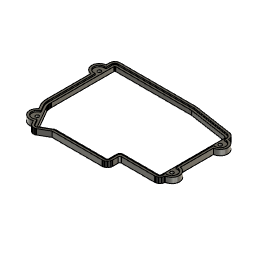
Lotus_case_v2 (Autodesk Fusion 360 design; units mm, degrees)
Autodesk Fusion 360 part; units mm, degrees
(part 1 of 2)
sketch "Sketch1" plane through (0, 0, 0) normal (0, 0, 1) x (1, 0, 0) in component "plate_left"
  circle A0 centre (76.6904, -49.9778) radius 4
  line L0 (80.5392, -30.7868) -> (81.5052, -30.6903)
  circle A1 centre (76.6904, -49.9778) radius 2
  line L1 (221.2947, -38.757) -> (223.044, -40.2889)
  circle A2 centre (86.1791, -132.9649) radius 2
  line L2 (81.5052, -30.6903) -> (172.0779, -30.687)
  line L3 (219.2863, -37.7893) -> (221.2947, -38.757)
  circle A3 centre (223.705, -53.9) radius 4
  circle A4 centre (223.705, -111.05) radius 2
  circle A5 centre (223.705, -111.05) radius 4
  circle A6 centre (223.705, -53.9) radius 2
  line L4 (172.0779, -30.687) -> (219.2863, -37.7893)
  line L5 (176.1036, -138.0502) -> (175.3059, -139.0179)
  line L6 (174.3382, -139.8156) -> (173.2321, -140.4142)
  line L7 (218.4, -126.194) -> (179.1936, -126.194)
  line L8 (99.2811, -148.0225) -> (98.1564, -148.3556)
  line L9 (224.5766, -121.0472) -> (224.2111, -122.2279)
  line L10 (76.6839, -118.0469) -> (76.2792, -116.505)
  line L11 (171.9999, -140.8) -> (170.9399, -140.905)
  line L12 (75.7005, -36.4881) -> (75.7987, -35.5252)
  line L13 (76.7158, -33.3442) -> (77.4564, -32.4462)
  line L14 (121.4, -62.05) -> (107.4, -62.05)
  line L15 (224.705, -119.9864) -> (224.5766, -121.0472)
  line L16 (173.2321, -140.4142) -> (171.9999, -140.8)
  line L17 (111.6629, -140.905) -> (99.9784, -147.6695)
  line L18 (76.2792, -116.505) -> (75.9418, -114.8181)
  line L19 (177.1936, -128.1938) -> (177.193, -134.6953)
  line L20 (99.9784, -147.6695) -> (99.2811, -148.0225)
  line L21 (75.7987, -35.5252) -> (76.1534, -34.3806)
  line L22 (77.4564, -32.4462) -> (78.3553, -31.7047)
  line L23 (121.4, -76.05) -> (121.4, -62.05)
  line L24 (130.85, -119.2) -> (116.85, -119.2)
  line L25 (223.044, -40.2889) -> (224.1387, -42.1727)
  line L26 (170.9399, -140.905) -> (111.6629, -140.905)
  line L27 (116.85, -119.2) -> (116.85, -133.2)
  line L28 (94.0822, -147.5328) -> (93.1049, -146.6975)
  line L29 (224.1387, -42.1727) -> (224.705, -44.1568)
  line L30 (107.4, -57) -> (121.4, -57)
  line L31 (121.4, -57) -> (121.4, -43)
  line L32 (176.7022, -136.9441) -> (176.1036, -138.0502)
  line L33 (75.7886, -113.0573) -> (75.7186, -112.1461)
  line L34 (75.7186, -112.1461) -> (75.6449, -110.7467)
  line L35 (116.85, -133.2) -> (130.85, -133.2)
  line L36 (107.4, -76.05) -> (121.4, -76.05)
  line L37 (98.23, -71.09) -> (98.23, -40.39)
  line L38 (223.6086, -123.3412) -> (222.8109, -124.3089)
  line L39 (177.082, -135.7313) -> (176.7022, -136.9441)
  line L40 (96.7866, -148.4476) -> (95.3567, -148.1592)
  line L41 (95.3567, -148.1592) -> (94.0822, -147.5328)
  line L42 (220.7348, -125.7064) -> (219.4745, -126.0997)
  line L43 (75.9418, -114.8181) -> (75.7886, -113.0573)
  line L44 (221.8432, -125.1066) -> (220.7348, -125.7064)
  line L45 (76.1534, -34.3806) -> (76.7158, -33.3442)
  line L46 (107.4, -43) -> (107.4, -57)
  line L47 (98.23, -40.39) -> (85.03, -40.39)
  line L48 (224.2111, -122.2279) -> (223.6086, -123.3412)
  line L49 (222.8109, -124.3089) -> (221.8432, -125.1066)
  line L50 (93.1049, -146.6975) -> (92.4734, -145.8895)
  line L51 (77.5111, -119.9268) -> (76.6839, -118.0469)
  line L52 (175.3059, -139.0179) -> (174.3382, -139.8156)
  line L53 (177.193, -134.6953) -> (177.082, -135.7313)
  line L54 (98.1564, -148.3556) -> (96.7866, -148.4476)
  line L55 (219.4745, -126.0997) -> (218.4, -126.194)
  line L56 (164.55, -97.75) -> (164.55, -111.75)
  line L57 (159.5, -77.31) -> (145.5, -77.31)
  line L58 (178.55, -54.6) -> (178.55, -40.6)
  line L59 (140.45, -73.65) -> (140.45, -59.65)
  line L60 (216.65, -99) -> (216.65, -85)
  line L61 (164.55, -111.75) -> (178.55, -111.75)
  line L62 (107.4, -100.15) -> (107.4, -114.15)
  line L63 (135.898, -117.828) -> (135.898, -131.828)
  line L64 (121.4, -114.15) -> (121.4, -100.15)
  line L65 (140.45, -40.6) -> (126.45, -40.6)
  line L66 (202.65, -99) -> (216.65, -99)
  line L67 (216.65, -60.9) -> (216.65, -46.9)
  line L68 (140.45, -78.7) -> (126.45, -78.7)
  line L69 (145.5, -72.26) -> (159.5, -72.26)
  line L70 (178.55, -111.75) -> (178.55, -97.75)
  line L71 (164.55, -73.65) -> (178.55, -73.65)
  line L72 (85.03, -71.09) -> (98.23, -71.09)
  line L73 (140.45, -54.6) -> (140.45, -40.6)
  line L74 (145.5, -91.31) -> (159.5, -91.31)
  line L75 (159.5, -72.26) -> (159.5, -58.26)
  line L76 (159.5, -58.26) -> (145.5, -58.26)
  line L77 (130.85, -133.2) -> (130.85, -119.2)
  line L78 (216.65, -46.9) -> (202.65, -46.9)
  line L79 (126.45, -40.6) -> (126.45, -54.6)
  line L80 (197.6, -78.45) -> (197.6, -64.45)
  line L81 (216.65, -85) -> (202.65, -85)
  line L82 (202.65, -85) -> (202.65, -99)
  line L83 (121.4, -43) -> (107.4, -43)
  line L84 (178.55, -40.6) -> (164.55, -40.6)
  line L85 (197.6, -102.55) -> (183.6, -102.55)
  line L86 (183.6, -102.55) -> (183.6, -116.55)
  line L87 (85.03, -40.39) -> (85.03, -71.09)
  line L88 (159.5, -91.31) -> (159.5, -77.31)
  line L89 (178.55, -73.65) -> (178.55, -59.65)
  line L90 (126.45, -92.7) -> (140.45, -92.7)
  line L91 (126.45, -54.6) -> (140.45, -54.6)
  line L92 (145.5, -58.26) -> (145.5, -72.26)
  line L93 (135.898, -131.828) -> (149.898, -131.828)
  line L94 (164.55, -40.6) -> (164.55, -54.6)
  line L95 (83.4748, -105.2852) -> (97.4748, -105.2852)
  line L96 (202.65, -60.9) -> (216.65, -60.9)
  line L97 (183.6, -83.5) -> (183.6, -97.5)
  line L98 (140.45, -59.65) -> (126.45, -59.65)
  line L99 (164.55, -59.65) -> (164.55, -73.65)
  line L100 (145.5, -77.31) -> (145.5, -91.31)
  line L101 (183.6, -116.55) -> (197.6, -116.55)
  line L102 (183.6, -78.45) -> (197.6, -78.45)
  line L103 (126.45, -59.65) -> (126.45, -73.65)
  line L104 (183.6, -97.5) -> (197.6, -97.5)
  line L105 (197.6, -64.45) -> (183.6, -64.45)
  line L106 (97.4748, -105.2852) -> (97.4748, -91.2851)
  line L107 (197.6, -83.5) -> (183.6, -83.5)
  line L108 (83.4748, -91.2851) -> (83.4748, -105.2852)
  line L109 (183.6, -64.45) -> (183.6, -78.45)
  line L110 (178.55, -59.65) -> (164.55, -59.65)
  line L111 (140.45, -92.7) -> (140.45, -78.7)
  line L112 (197.6, -116.55) -> (197.6, -102.55)
  line L113 (126.45, -73.65) -> (140.45, -73.65)
  line L114 (149.898, -131.828) -> (149.898, -117.828)
  line L115 (107.4, -62.05) -> (107.4, -76.05)
  line L116 (149.898, -117.828) -> (135.898, -117.828)
  line L117 (202.65, -46.9) -> (202.65, -60.9)
  line L118 (178.55, -97.75) -> (164.55, -97.75)
  line L119 (107.4, -114.15) -> (121.4, -114.15)
  line L120 (121.4, -100.15) -> (107.4, -100.15)
  line L121 (197.6, -97.5) -> (197.6, -83.5)
  line L122 (145.5, -96.36) -> (145.5, -110.36)
  line L123 (164.55, -54.6) -> (178.55, -54.6)
  line L124 (145.5, -110.36) -> (159.5, -110.36)
  line L125 (126.45, -78.7) -> (126.45, -92.7)
  line L126 (79.3908, -31.1434) -> (80.5392, -30.7868)
  line L127 (78.3553, -31.7047) -> (79.3908, -31.1434)
  arc A7 (75.6971, -41.0327) -> (75.6837, -58.9213) centre (76.6904, -49.9778) ccw
  arc A8 (224.704, -119.9944) -> (224.705, -102.1057) centre (223.705, -111.05) ccw
  arc A9 (80.8467, -125.7147) -> (89.7788, -141.2137) centre (86.1791, -132.9649) ccw
  arc A10 (224.705, -62.8443) -> (224.705, -44.9557) centre (223.705, -53.9) ccw
  circle A11 centre (86.1791, -132.9649) radius 4
  line L128 (144.5, -92.31) -> (160.5, -92.31)
  line L129 (182.6, -98.5) -> (198.6, -98.5)
  line L130 (125.45, -93.7) -> (141.45, -93.7)
  line L131 (163.55, -58.65) -> (163.55, -74.65)
  line L132 (141.45, -77.7) -> (125.45, -77.7)
  line L133 (179.55, -77.7) -> (163.55, -77.7)
  line L134 (179.55, -58.65) -> (163.55, -58.65)
  line L135 (125.45, -77.7) -> (125.45, -93.7)
  line L136 (217.65, -100) -> (217.65, -84)
  line L137 (198.6, -63.45) -> (182.6, -63.45)
  line L138 (144.5, -76.31) -> (144.5, -92.31)
  line L139 (182.6, -79.45) -> (198.6, -79.45)
  line L140 (198.6, -82.5) -> (182.6, -82.5)
  line L141 (201.65, -80.95) -> (217.65, -80.95)
  line L142 (198.6, -79.45) -> (198.6, -63.45)
  line L143 (217.65, -119.05) -> (217.65, -103.05)
  line L144 (201.65, -103.05) -> (201.65, -119.05)
  line L145 (198.6, -101.55) -> (182.6, -101.55)
  line L146 (217.65, -64.95) -> (201.65, -64.95)
  line L147 (106.4, -96.1) -> (122.4, -96.1)
  line L148 (201.65, -84) -> (201.65, -100)
  line L149 (163.55, -74.65) -> (179.55, -74.65)
  line L150 (163.55, -93.7) -> (179.55, -93.7)
  line L151 (217.65, -80.95) -> (217.65, -64.95)
  line L152 (163.55, -112.75) -> (179.55, -112.75)
  line L153 (179.55, -74.65) -> (179.55, -58.65)
  line L154 (160.5, -92.31) -> (160.5, -76.31)
  line L155 (144.5, -95.36) -> (144.5, -111.36)
  line L156 (163.55, -96.75) -> (163.55, -112.75)
  line L157 (141.45, -96.75) -> (125.45, -96.75)
  line L158 (106.4, -80.1) -> (106.4, -96.1)
  line L159 (182.6, -63.45) -> (182.6, -79.45)
  line L160 (144.5, -111.36) -> (160.5, -111.36)
  line L161 (198.6, -117.55) -> (198.6, -101.55)
  line L162 (217.65, -103.05) -> (201.65, -103.05)
  line L163 (125.45, -96.75) -> (125.45, -112.75)
  line L164 (125.45, -112.75) -> (141.45, -112.75)
  line L165 (201.65, -119.05) -> (217.65, -119.05)
  line L166 (160.5, -76.31) -> (144.5, -76.31)
  line L167 (160.5, -73.26) -> (160.5, -57.26)
  line L168 (201.65, -100) -> (217.65, -100)
  line L169 (106.4, -115.15) -> (122.4, -115.15)
  line L170 (198.6, -98.5) -> (198.6, -82.5)
  line L171 (217.65, -84) -> (201.65, -84)
  line L172 (179.55, -96.75) -> (163.55, -96.75)
  line L173 (122.4, -80.1) -> (106.4, -80.1)
  line L174 (182.6, -117.55) -> (198.6, -117.55)
  line L175 (122.4, -115.15) -> (122.4, -99.15)
  line L176 (97.4748, -91.2851) -> (83.4748, -91.2851)
  line L177 (80.7003, -36.7444) -> (80.7223, -36.5288)
  line L178 (80.645, -110.617) -> (80.7003, -36.7444)
  line L179 (97.4269, -143.357) -> (97.2682, -143.404)
  line L180 (164.55, -92.7) -> (178.55, -92.7)
  line L181 (80.7834, -36.3316) -> (80.8802, -36.1532)
  line L182 (219.705, -119.685) -> (219.667, -119.999)
  line L183 (159.5, -110.36) -> (159.5, -96.36)
  line L184 (219.442, -120.535) -> (219.259, -120.757)
  line L185 (80.7223, -36.5288) -> (80.7834, -36.3316)
  line L186 (173.244, -122.218) -> (172.817, -122.736)
  line L187 (219.58, -120.28) -> (219.442, -120.535)
  line L188 (178.55, -92.7) -> (178.55, -78.7)
  line L189 (171.704, -35.687) -> (217.796, -42.6214)
  line L190 (97.5948, -143.272) -> (97.4269, -143.357)
  line L191 (140.45, -97.75) -> (126.45, -97.75)
  line L192 (97.2682, -143.404) -> (97.1193, -143.414)
  line L193 (171.532, -135.649) -> (171.277, -135.787)
  line L194 (96.8523, -143.323) -> (96.7353, -143.223)
  line L195 (81.153, -115.379) -> (80.899, -114.109)
  line L196 (81.5392, -35.7118) -> (81.7544, -35.6903)
  line L197 (80.899, -114.109) -> (80.772, -112.649)
  line L198 (80.8802, -36.1532) -> (81.0083, -35.9979)
  line L199 (219.133, -43.5102) -> (219.502, -44.1452)
  line L200 (171.277, -135.787) -> (170.996, -135.875)
  line L201 (140.45, -111.75) -> (140.45, -97.75)
  line L202 (218.512, -42.9664) -> (219.133, -43.5102)
  line L203 (217.796, -42.6214) -> (218.512, -42.9664)
  line L204 (126.45, -97.75) -> (126.45, -111.75)
  line L205 (80.7085, -111.823) -> (80.645, -110.617)
  line L206 (81.0083, -35.9979) -> (81.1637, -35.8697)
  line L207 (219.705, -44.8564) -> (219.705, -119.685)
  line L208 (96.9805, -143.386) -> (96.8523, -143.323)
  line L209 (170.693, -135.905) -> (110.32, -135.905)
  line L210 (219.667, -119.999) -> (219.58, -120.28)
  line L211 (219.037, -120.94) -> (218.782, -121.078)
  line L212 (171.937, -135.244) -> (171.754, -135.466)
  line L213 (97.1193, -143.414) -> (96.9805, -143.386)
  line L214 (80.772, -112.649) -> (80.7085, -111.823)
  line L215 (81.9785, -117.665) -> (81.4197, -116.395)
  line L216 (96.7353, -143.223) -> (96.6298, -143.088)
  line L217 (178.55, -78.7) -> (164.55, -78.7)
  line L218 (216.65, -79.95) -> (216.65, -65.95)
  line L219 (81.1637, -35.8697) -> (81.3421, -35.773)
  line L220 (218.782, -121.078) -> (218.5, -121.166)
  line L221 (218.5, -121.166) -> (218.181, -121.194)
  line L222 (175.719, -121.194) -> (175.014, -121.265)
  line L223 (96.6298, -143.088) -> (81.9785, -117.665)
  line L224 (171.754, -135.466) -> (171.532, -135.649)
  line L225 (175.014, -121.265) -> (174.356, -121.468)
  line L226 (218.181, -121.194) -> (175.719, -121.194)
  line L227 (81.3421, -35.773) -> (81.5392, -35.7118)
  line L228 (219.259, -120.757) -> (219.037, -120.94)
  line L229 (110.32, -135.905) -> (97.5948, -143.272)
  line L230 (202.65, -79.95) -> (216.65, -79.95)
  line L231 (219.502, -44.1452) -> (219.705, -44.8564)
  line L232 (126.45, -111.75) -> (140.45, -111.75)
  line L233 (170.996, -135.875) -> (170.693, -135.905)
  line L234 (173.762, -121.791) -> (173.244, -122.218)
  line L235 (174.356, -121.468) -> (173.762, -121.791)
  line L236 (202.65, -65.95) -> (202.65, -79.95)
  line L237 (164.55, -78.7) -> (164.55, -92.7)
  line L238 (216.65, -65.95) -> (202.65, -65.95)
  line L239 (159.5, -96.36) -> (145.5, -96.36)
  line L240 (81.7544, -35.6903) -> (171.704, -35.687)
  line L241 (81.4197, -116.395) -> (81.153, -115.379)
  line L242 (163.55, -55.6) -> (179.55, -55.6)
  line L243 (107.4, -81.1) -> (107.4, -95.1)
  line L244 (106.4, -42) -> (106.4, -58)
  line L245 (145.5, -39.21) -> (145.5, -53.21)
  line L246 (217.65, -61.9) -> (217.65, -45.9)
  line L247 (95.609, -135.6097) -> (107.7334, -128.6097)
  line L248 (159.5, -53.21) -> (159.5, -39.21)
  line L249 (141.45, -58.65) -> (125.45, -58.65)
  line L250 (160.5, -38.21) -> (144.5, -38.21)
  line L251 (172.817, -122.736) -> (172.494, -123.331)
  line L252 (179.55, -39.6) -> (163.55, -39.6)
  line L253 (182.6, -60.4) -> (198.6, -60.4)
  line L254 (198.6, -60.4) -> (198.6, -44.4)
  line L255 (122.4, -58) -> (122.4, -42)
  line L256 (172.075, -134.989) -> (171.937, -135.244)
  line L257 (125.45, -74.65) -> (141.45, -74.65)
  line L258 (183.6, -59.4) -> (197.6, -59.4)
  line L259 (125.45, -58.65) -> (125.45, -74.65)
  line L260 (144.5, -38.21) -> (144.5, -54.21)
  line L261 (172.29, -123.988) -> (172.194, -124.696)
  line L262 (100.7334, -116.4853) -> (88.609, -123.4853)
  line L263 (172.494, -123.331) -> (172.29, -123.988)
  line L264 (201.65, -45.9) -> (201.65, -61.9)
  line L265 (144.5, -73.26) -> (160.5, -73.26)
  line L266 (122.4, -61.05) -> (106.4, -61.05)
  line L267 (106.4, -61.05) -> (106.4, -77.05)
  line L268 (216.65, -118.05) -> (216.65, -104.05)
  line L269 (122.4, -42) -> (106.4, -42)
  line L270 (121.4, -81.1) -> (107.4, -81.1)
  line L271 (197.6, -45.4) -> (183.6, -45.4)
  line L272 (125.45, -55.6) -> (141.45, -55.6)
  line L273 (183.6, -45.4) -> (183.6, -59.4)
  line L274 (160.5, -54.21) -> (160.5, -38.21)
  line L275 (154.95, -130.8) -> (168.95, -130.8)
  line L276 (197.6, -59.4) -> (197.6, -45.4)
  line L277 (107.7334, -128.6097) -> (100.7334, -116.4853)
  line L278 (121.4, -95.1) -> (121.4, -81.1)
  line L279 (106.4, -58) -> (122.4, -58)
  line L280 (202.65, -118.05) -> (216.65, -118.05)
  line L281 (216.65, -104.05) -> (202.65, -104.05)
  line L282 (141.45, -39.6) -> (125.45, -39.6)
  line L283 (125.45, -39.6) -> (125.45, -55.6)
  line L284 (202.65, -104.05) -> (202.65, -118.05)
  line L285 (172.194, -124.696) -> (172.193, -134.428)
  line L286 (122.4, -77.05) -> (122.4, -61.05)
  line L287 (163.55, -39.6) -> (163.55, -55.6)
  line L288 (179.55, -55.6) -> (179.55, -39.6)
  line L289 (217.65, -45.9) -> (201.65, -45.9)
  line L290 (141.45, -55.6) -> (141.45, -39.6)
  line L291 (198.6, -44.4) -> (182.6, -44.4)
  line L292 (141.45, -74.65) -> (141.45, -58.65)
  line L293 (168.95, -130.8) -> (168.95, -116.8)
  line L294 (145.5, -53.21) -> (159.5, -53.21)
  line L295 (154.95, -116.8) -> (154.95, -130.8)
  line L296 (168.95, -116.8) -> (154.95, -116.8)
  line L297 (182.6, -44.4) -> (182.6, -60.4)
  line L298 (144.5, -54.21) -> (160.5, -54.21)
  line L299 (122.4, -96.1) -> (122.4, -80.1)
  line L300 (159.5, -39.21) -> (145.5, -39.21)
  line L301 (88.609, -123.4853) -> (95.609, -135.6097)
  line L302 (172.193, -134.428) -> (172.163, -134.708)
  line L303 (106.4, -77.05) -> (122.4, -77.05)
  line L304 (201.65, -61.9) -> (217.65, -61.9)
  line L305 (107.4, -95.1) -> (121.4, -95.1)
  line L306 (172.163, -134.708) -> (172.075, -134.989)
  line L307 (160.5, -95.36) -> (144.5, -95.36)
  line L308 (141.45, -112.75) -> (141.45, -96.75)
  line L309 (122.4, -99.15) -> (106.4, -99.15)
  line L310 (160.5, -57.26) -> (144.5, -57.26)
  line L311 (201.65, -64.95) -> (201.65, -80.95)
  line L312 (179.55, -93.7) -> (179.55, -77.7)
  line L313 (179.55, -112.75) -> (179.55, -96.75)
  line L314 (144.5, -57.26) -> (144.5, -73.26)
  line L315 (106.4, -99.15) -> (106.4, -115.15)
  line L316 (182.6, -82.5) -> (182.6, -98.5)
  line L317 (182.6, -101.55) -> (182.6, -117.55)
  line L318 (163.55, -77.7) -> (163.55, -93.7)
  line L319 (141.45, -93.7) -> (141.45, -77.7)
  line L320 (82.4748, -106.2852) -> (98.4748, -106.2852)
  line L321 (160.5, -111.36) -> (160.5, -95.36)
  line L322 (95.23, -68.09) -> (95.23, -43.39)
  line L323 (88.03, -43.39) -> (88.03, -68.09)
  line L324 (169.95, -131.8) -> (169.95, -115.8)
  line L325 (82.4748, -90.2851) -> (82.4748, -106.2852)
  line L326 (131.85, -134.2) -> (131.85, -118.2)
  line L327 (115.85, -134.2) -> (131.85, -134.2)
  line L328 (115.85, -118.2) -> (115.85, -134.2)
  line L329 (87.243, -123.1193) -> (95.243, -136.9757)
  line L330 (150.898, -132.828) -> (150.898, -116.828)
  line L331 (95.243, -136.9757) -> (109.0994, -128.9757)
  line L332 (150.898, -116.828) -> (134.898, -116.828)
  line L333 (98.4748, -90.2851) -> (82.4748, -90.2851)
  line L334 (131.85, -118.2) -> (115.85, -118.2)
  line L335 (98.4748, -106.2852) -> (98.4748, -90.2851)
  line L336 (169.95, -115.8) -> (153.95, -115.8)
  line L337 (153.95, -131.8) -> (169.95, -131.8)
  line L338 (153.95, -115.8) -> (153.95, -131.8)
  line L339 (88.03, -68.09) -> (95.23, -68.09)
  line L340 (134.898, -132.828) -> (150.898, -132.828)
  line L341 (101.0994, -115.1193) -> (87.243, -123.1193)
  line L342 (134.898, -116.828) -> (134.898, -132.828)
  line L343 (109.0994, -128.9757) -> (101.0994, -115.1193)
  line L344 (95.23, -43.39) -> (88.03, -43.39)
  line L345 (218.5412, -40.2054) -> (219.9033, -40.8617)
  line L346 (219.9033, -40.8617) -> (221.0885, -41.8996)
  line L347 (221.0885, -41.8996) -> (221.8203, -43.1589)
  line L348 (221.8203, -43.1589) -> (222.205, -44.5066)
  line L349 (222.205, -119.8357) -> (222.1218, -120.5231)
  line L350 (222.1218, -120.5231) -> (221.8955, -121.2539)
  line L351 (221.8955, -121.2539) -> (221.5253, -121.9381)
  line L352 (221.5253, -121.9381) -> (221.0349, -122.5329)
  line L353 (221.0349, -122.5329) -> (220.4401, -123.0233)
  line L354 (220.4401, -123.0233) -> (219.7584, -123.3922)
  line L355 (219.7584, -123.3922) -> (218.9873, -123.6328)
  line L356 (218.9873, -123.6328) -> (218.2905, -123.694)
  line L357 (218.2905, -123.694) -> (177.6938, -123.694)
  line L358 (174.6938, -126.6937) -> (174.693, -134.5617)
  line L359 (174.693, -134.5617) -> (174.6225, -135.2197)
  line L360 (174.6225, -135.2197) -> (174.3886, -135.9665)
  line L361 (174.3886, -135.9665) -> (174.0203, -136.6471)
  line L362 (174.0203, -136.6471) -> (173.5299, -137.2419)
  line L363 (173.5299, -137.2419) -> (172.9351, -137.7323)
  line L364 (172.9351, -137.7323) -> (172.2545, -138.1006)
  line L365 (172.2545, -138.1006) -> (171.498, -138.3375)
  line L366 (171.498, -138.3375) -> (170.8165, -138.405)
  line L367 (170.8165, -138.405) -> (110.9915, -138.405)
  line L368 (110.9915, -138.405) -> (98.7866, -145.4708)
  line L369 (98.7866, -145.4708) -> (98.354, -145.6898)
  line L370 (98.354, -145.6898) -> (97.7123, -145.8798)
  line L371 (97.7123, -145.8798) -> (96.953, -145.9308)
  line L372 (96.953, -145.9308) -> (96.1686, -145.7726)
  line L373 (96.1686, -145.7726) -> (95.4672, -145.4279)
  line L374 (95.4672, -145.4279) -> (94.9201, -144.9603)
  line L375 (94.9201, -144.9603) -> (94.5516, -144.4887)
  line L376 (79.7448, -118.7959) -> (79.0518, -117.2209)
  line L377 (79.0518, -117.2209) -> (78.7161, -115.942)
  line L378 (78.7161, -115.942) -> (78.4204, -114.4636)
  line L379 (78.4204, -114.4636) -> (78.2803, -112.8531)
  line L380 (78.2803, -112.8531) -> (78.2135, -111.9846)
  line L381 (78.2135, -111.9846) -> (78.145, -110.6818)
  line L382 (78.2004, -36.6162) -> (78.2605, -36.027)
  line L383 (78.2605, -36.027) -> (78.4684, -35.3561)
  line L384 (78.4684, -35.3561) -> (78.798, -34.7487)
  line L385 (78.798, -34.7487) -> (79.2324, -34.2221)
  line L386 (79.2324, -34.2221) -> (79.7595, -33.7872)
  line L387 (79.7595, -33.7872) -> (80.3665, -33.4582)
  line L388 (80.3665, -33.4582) -> (81.0392, -33.2493)
  line L389 (81.0392, -33.2493) -> (81.6298, -33.1903)
  line L390 (81.6298, -33.1903) -> (171.891, -33.187)
  line L391 (171.891, -33.187) -> (218.5412, -40.2054)
  arc A12 (78.1951, -43.6543) -> (78.1857, -56.3034) centre (76.6904, -49.9778) ccw
  line L392 (78.1951, -43.6543) -> (78.2004, -36.6162)
  line L393 (75.6971, -41.0327) -> (75.7005, -36.4881)
  line L394 (78.145, -110.6818) -> (78.1857, -56.3034)
  line L395 (75.6449, -110.7467) -> (75.6837, -58.9213)
  arc A13 (84.3208, -126.7362) -> (90.6367, -137.6956) centre (86.1791, -132.9649) ccw
  line L396 (94.5516, -144.4887) -> (90.6367, -137.6956)
  line L397 (84.3208, -126.7362) -> (79.7448, -118.7959)
  line L398 (80.8467, -125.7147) -> (77.5111, -119.9268)
  line L399 (92.4734, -145.8895) -> (89.7788, -141.2137)
  arc A14 (222.205, -117.3746) -> (222.205, -104.7254) centre (223.705, -111.05) ccw
  line L400 (222.205, -117.3746) -> (222.205, -119.8357)
  line L401 (224.705, -62.8443) -> (224.705, -102.1057)
  line L402 (224.705, -44.1568) -> (224.705, -44.9557)
  arc A15 (222.205, -60.2246) -> (222.205, -47.5754) centre (223.705, -53.9) ccw
  line L403 (222.205, -60.2246) -> (222.205, -104.7254)
  line L404 (222.205, -44.5066) -> (222.205, -47.5754)
  arc A16 (179.1936, -126.194) -> (177.1936, -128.1938) centre (179.1936, -128.194) ccw
  arc A17 (177.6938, -123.694) -> (174.6938, -126.6937) centre (177.6938, -126.694) ccw
  dimension "d6" = 13
  dimension "d7" = 13
  dimension "d8" = 13
  dimension "d9" = 13
  dimension "d10" = 2
  dimension "d11" = 3
  constraint concentric A1 A12
  constraint concentric A11 A13
  constraint concentric A5 A14
  constraint concentric A10 A15
  constraint coincident A12.start L394
  constraint collinear L392 L394
  constraint collinear L393 L395
  constraint coincident A13.start L396
  constraint collinear L396 L397
  constraint collinear L398 L399
  constraint coincident A14.start L404
  constraint collinear L400 L404
  constraint collinear L401 L402
  constraint coincident A15.start L404
  constraint collinear L403 L404
  constraint tangent L19 A16
  constraint tangent L7 A16
  constraint tangent L358 A17
  constraint tangent L357 A17
  measures "d6" diameter of A12
  measures "d7" diameter of A13
  measures "d8" diameter of A14
  measures "d9" diameter of A15
  measures "d10" radius of A16
  measures "d11" radius of A17
form "Form1" [no effect] in component "plate_left"
extrude "Extrude1" add sketch "Sketch1" along normal blind 3 contours A0 | L177 L178 L179 L181 L182 L184 L185 L186 L187 L189 L190 L192 L193 L194 L195 L196 L197 L198 L199 L200 L202 L203 L205 L206 L207 L208 L209 L210 L211 L212 L213 L214 L215 L216 L219 L220 L221 L222 L223 L224 L225 L226 L227 L228 L229 L231 L233 L234 L235 L240 L241 L251 L256 L261 L263 L285 L302 L306 | A3 | A5 | A11 | L0 L1 L2 L3 L4 L5 L6 L7 L8 L9 L10 L11 L12 L13 L15 L16 L17 L18 L19 L20 L21 L22 L25 L26 L28 L29 L32 L33 L34 L38 L39 L40 L41 L42 L43 L44 L45 L48 L49 L50 L51 L52 L53 L54 L55 L126 L127 A7 A8 A9 A10 L393 L395 L398 L399 L401 L402 A16 | L345 L346 L347 L348 L349 L350 L351 L352 L353 L354 L355 L356 L357 L358 L359 L360 L361 L362 L363 L364 L365 L366 L367 L368 L369 L370 L371 L372 L373 L374 L375 L376 L377 L378 L379 L380 L381 L382 L383 L384 L385 L386 L387 L388 L389 L390 L391 A12 L392 L394 A13 L396 L397 A14 L400 A15 L403 L404 A17 makes body 1 in component "plate_left"
extrude "Extrude2" add sketch "Sketch1" along normal blind 1.5 contours L37 L47 L72 L87 | L128 L138 L154 L166 | L129 L140 L170 L316 | L130 L132 L135 L319 | L131 L134 L149 L153 | L133 L150 L312 L318 | L136 L148 L168 L171 | L137 L139 L142 L159 | L141 L146 L151 L311 | L143 L144 L162 L165 | L145 L161 L174 L317 | L147 L158 L173 L299 | L152 L156 L172 L313 | L155 L160 L307 L321 | L157 L163 L164 L308 | L167 L265 L310 L314 | L169 L175 L309 L315 | L242 L252 L287 L288 | L244 L255 L269 L279 | L246 L264 L289 L304 | L249 L257 L259 L292 | L250 L260 L274 L298 | L253 L254 L291 L297 | L266 L267 L286 L303 | L272 L282 L283 L290 | L320 L325 L333 L335 | L324 L336 L337 L338 | L326 L327 L328 L334 | L329 L331 L341 L343 | L330 L332 L340 L342 bodies 1 in component "plate_left"
extrude "Extrude3" cut sketch "Sketch1" along normal blind 3 contours L0 L1 L2 L3 L4 L5 L6 L7 L8 L9 L10 L11 L12 L13 L15 L16 L17 L18 L19 L20 L21 L22 L25 L26 L28 L29 L32 L33 L34 L38 L39 L40 L41 L42 L43 L44 L45 L48 L49 L50 L51 L52 L53 L54 L55 L126 L127 A7 A8 A9 A10 L393 L395 L398 L399 L401 L402 A16 bodies 1 in component "plate_left"
sketch "clean_plate_v4.1" plane through (0, 0, 0) normal (0, 0, 1) x (1, 0, 0) in component "bottom_right"
  line L0 (78.2605, -36.027) -> (78.4684, -35.3561)
  line L1 (81.0392, -33.2493) -> (81.6298, -33.1903)
  line L2 (78.4684, -35.3561) -> (78.798, -34.7487)
  line L3 (171.891, -33.187) -> (218.5412, -40.2054)
  line L4 (78.2004, -36.6162) -> (78.2605, -36.027)
  line L5 (78.798, -34.7487) -> (79.2324, -34.2221)
  line L6 (75.6449, -110.7467) -> (75.6837, -58.9213)
  line L7 (224.705, -44.1568) -> (224.705, -44.9557)
  arc A0 (78.1857, -56.3034) -> (78.1951, -43.6543) centre (76.6904, -49.9778) cw
  line L8 (82.4748, -106.2852) -> (98.4748, -106.2852)
  line L9 (98.4748, -90.2851) -> (82.4748, -90.2851)
  line L10 (168.95, -116.8) -> (154.95, -116.8)
  line L11 (125.45, -39.6) -> (125.45, -55.6)
  line L12 (154.95, -130.8) -> (168.95, -130.8)
  line L13 (95.23, -43.39) -> (88.03, -43.39)
  line L14 (95.23, -68.09) -> (95.23, -43.39)
  line L15 (98.4748, -106.2852) -> (98.4748, -90.2851)
  line L16 (202.65, -104.05) -> (202.65, -118.05)
  line L17 (154.95, -116.8) -> (154.95, -130.8)
  line L18 (216.65, -118.05) -> (216.65, -104.05)
  line L19 (216.65, -104.05) -> (202.65, -104.05)
  line L20 (122.4, -77.05) -> (122.4, -61.05)
  line L21 (168.95, -130.8) -> (168.95, -116.8)
  line L22 (202.65, -118.05) -> (216.65, -118.05)
  line L23 (141.45, -39.6) -> (125.45, -39.6)
  line L24 (141.45, -55.6) -> (141.45, -39.6)
  line L25 (125.45, -55.6) -> (141.45, -55.6)
  line L26 (216.65, -79.95) -> (216.65, -65.95)
  line L27 (82.4748, -90.2851) -> (82.4748, -106.2852)
  line L28 (80.8467, -125.7147) -> (77.5111, -119.9268)
  line L29 (78.1951, -43.6543) -> (78.2004, -36.6162)
  line L30 (79.7595, -33.7872) -> (80.3665, -33.4582)
  line L31 (224.705, -62.8443) -> (224.705, -102.1057)
  line L32 (75.6971, -41.0327) -> (75.7005, -36.4881)
  line L33 (171.498, -138.3375) -> (170.8165, -138.405)
  line L34 (170.8165, -138.405) -> (110.9915, -138.405)
  line L35 (87.243, -123.1193) -> (95.243, -136.9757)
  line L36 (222.205, -60.2246) -> (222.205, -104.7254)
  line L37 (115.85, -118.2) -> (115.85, -134.2)
  line L38 (150.898, -132.828) -> (150.898, -116.828)
  line L39 (174.0203, -136.6471) -> (173.5299, -137.2419)
  line L40 (78.145, -110.6818) -> (78.1857, -56.3034)
  line L41 (92.4734, -145.8895) -> (89.7788, -141.2137)
  line L42 (79.2324, -34.2221) -> (79.7595, -33.7872)
  arc A1 (179.1936, -126.194) -> (177.1936, -128.1938) centre (179.1936, -128.194) ccw
  line L43 (80.3665, -33.4582) -> (81.0392, -33.2493)
  line L44 (81.6298, -33.1903) -> (171.891, -33.187)
  line L45 (131.85, -118.2) -> (115.85, -118.2)
  line L46 (222.205, -119.8357) -> (222.1218, -120.5231)
  line L47 (169.95, -115.8) -> (153.95, -115.8)
  line L48 (153.95, -131.8) -> (169.95, -131.8)
  line L49 (115.85, -134.2) -> (131.85, -134.2)
  line L50 (222.205, -117.3746) -> (222.205, -119.8357)
  line L51 (220.4401, -123.0233) -> (219.7584, -123.3922)
  line L52 (219.7584, -123.3922) -> (218.9873, -123.6328)
  line L53 (174.6225, -135.2197) -> (174.3886, -135.9665)
  line L54 (221.8203, -43.1589) -> (222.205, -44.5066)
  arc A2 (222.205, -104.7254) -> (222.205, -117.3746) centre (223.705, -111.05) cw
  line L55 (134.898, -116.828) -> (134.898, -132.828)
  line L56 (169.95, -131.8) -> (169.95, -115.8)
  line L57 (163.55, -77.7) -> (163.55, -93.7)
  line L58 (197.6, -83.5) -> (183.6, -83.5)
  line L59 (197.6, -102.55) -> (183.6, -102.55)
  line L60 (141.45, -77.7) -> (125.45, -77.7)
  line L61 (198.6, -98.5) -> (198.6, -82.5)
  line L62 (179.55, -58.65) -> (163.55, -58.65)
  line L63 (183.6, -78.45) -> (197.6, -78.45)
  line L64 (78.3553, -31.7047) -> (79.3908, -31.1434)
  line L65 (198.6, -82.5) -> (182.6, -82.5)
  line L66 (159.5, -96.36) -> (145.5, -96.36)
  line L67 (217.65, -84) -> (201.65, -84)
  line L68 (125.45, -93.7) -> (141.45, -93.7)
  line L69 (163.55, -74.65) -> (179.55, -74.65)
  line L70 (201.65, -100) -> (217.65, -100)
  circle A3 centre (86.1791, -132.9649) radius 4
  line L71 (182.6, -63.45) -> (182.6, -79.45)
  line L72 (79.3908, -31.1434) -> (80.5392, -30.7868)
  line L73 (145.5, -110.36) -> (159.5, -110.36)
  line L74 (179.55, -93.7) -> (179.55, -77.7)
  line L75 (198.6, -79.45) -> (198.6, -63.45)
  line L76 (217.65, -80.95) -> (217.65, -64.95)
  line L77 (179.55, -77.7) -> (163.55, -77.7)
  line L78 (217.65, -64.95) -> (201.65, -64.95)
  line L79 (201.65, -84) -> (201.65, -100)
  line L80 (179.55, -74.65) -> (179.55, -58.65)
  line L81 (183.6, -97.5) -> (197.6, -97.5)
  line L82 (159.5, -110.36) -> (159.5, -96.36)
  line L83 (201.65, -64.95) -> (201.65, -80.95)
  line L84 (217.65, -103.05) -> (201.65, -103.05)
  line L85 (217.65, -100) -> (217.65, -84)
  line L86 (201.65, -103.05) -> (201.65, -119.05)
  line L87 (201.65, -119.05) -> (217.65, -119.05)
  line L88 (198.6, -63.45) -> (182.6, -63.45)
  line L89 (198.6, -101.55) -> (182.6, -101.55)
  line L90 (217.65, -119.05) -> (217.65, -103.05)
  line L91 (125.45, -77.7) -> (125.45, -93.7)
  line L92 (182.6, -101.55) -> (182.6, -117.55)
  arc A4 (224.705, -62.8443) -> (224.705, -44.9557) centre (223.705, -53.9) ccw
  line L93 (163.55, -55.6) -> (179.55, -55.6)
  line L94 (179.55, -39.6) -> (163.55, -39.6)
  line L95 (144.5, -54.21) -> (160.5, -54.21)
  line L96 (88.609, -123.4853) -> (95.609, -135.6097)
  line L97 (202.65, -65.95) -> (202.65, -79.95)
  line L98 (121.4, -81.1) -> (107.4, -81.1)
  line L99 (107.4, -95.1) -> (121.4, -95.1)
  line L100 (122.4, -58) -> (122.4, -42)
  line L101 (201.65, -45.9) -> (201.65, -61.9)
  line L102 (107.4, -81.1) -> (107.4, -95.1)
  line L103 (179.55, -55.6) -> (179.55, -39.6)
  line L104 (163.55, -39.6) -> (163.55, -55.6)
  line L105 (145.5, -39.21) -> (145.5, -53.21)
  line L106 (107.7334, -128.6097) -> (100.7334, -116.4853)
  line L107 (159.5, -39.21) -> (145.5, -39.21)
  line L108 (106.4, -58) -> (122.4, -58)
  line L109 (141.45, -58.65) -> (125.45, -58.65)
  line L110 (145.5, -53.21) -> (159.5, -53.21)
  line L111 (106.4, -42) -> (106.4, -58)
  line L112 (201.65, -61.9) -> (217.65, -61.9)
  line L113 (95.609, -135.6097) -> (107.7334, -128.6097)
  line L114 (159.5, -53.21) -> (159.5, -39.21)
  line L115 (216.65, -65.95) -> (202.65, -65.95)
  line L116 (100.7334, -116.4853) -> (88.609, -123.4853)
  line L117 (121.4, -95.1) -> (121.4, -81.1)
  line L118 (122.4, -42) -> (106.4, -42)
  line L119 (198.6, -60.4) -> (198.6, -44.4)
  line L120 (202.65, -79.95) -> (216.65, -79.95)
  line L121 (217.65, -61.9) -> (217.65, -45.9)
  line L122 (217.65, -45.9) -> (201.65, -45.9)
  line L123 (182.6, -60.4) -> (198.6, -60.4)
  line L124 (174.3382, -139.8156) -> (173.2321, -140.4142)
  line L125 (107.4, -76.05) -> (121.4, -76.05)
  line L126 (80.5392, -30.7868) -> (81.5052, -30.6903)
  line L127 (122.4, -61.05) -> (106.4, -61.05)
  line L128 (125.45, -58.65) -> (125.45, -74.65)
  line L129 (160.5, -38.21) -> (144.5, -38.21)
  line L130 (160.5, -54.21) -> (160.5, -38.21)
  line L131 (221.2947, -38.757) -> (223.044, -40.2889)
  circle A5 centre (223.705, -111.05) radius 4
  line L132 (182.6, -44.4) -> (182.6, -60.4)
  circle A6 centre (86.1791, -132.9649) radius 2
  line L133 (224.705, -119.9864) -> (224.5766, -121.0472)
  line L134 (121.4, -76.05) -> (121.4, -62.05)
  line L135 (173.2321, -140.4142) -> (171.9999, -140.8)
  line L136 (76.2792, -116.505) -> (75.9418, -114.8181)
  line L137 (141.45, -74.65) -> (141.45, -58.65)
  line L138 (197.6, -59.4) -> (197.6, -45.4)
  circle A7 centre (223.705, -53.9) radius 4
  line L139 (144.5, -38.21) -> (144.5, -54.21)
  line L140 (198.6, -44.4) -> (182.6, -44.4)
  circle A8 centre (223.705, -53.9) radius 2
  line L141 (219.2863, -37.7893) -> (221.2947, -38.757)
  line L142 (111.6629, -140.905) -> (99.9784, -147.6695)
  line L143 (176.1036, -138.0502) -> (175.3059, -139.0179)
  line L144 (177.1936, -128.1938) -> (177.193, -134.6953)
  line L145 (140.45, -111.75) -> (140.45, -97.75)
  line L146 (126.45, -97.75) -> (126.45, -111.75)
  circle A9 centre (76.6904, -49.9778) radius 4
  circle A10 centre (223.705, -111.05) radius 2
  line L147 (183.6, -45.4) -> (183.6, -59.4)
  line L148 (106.4, -77.05) -> (122.4, -77.05)
  line L149 (126.45, -111.75) -> (140.45, -111.75)
  line L150 (197.6, -45.4) -> (183.6, -45.4)
  line L151 (172.0779, -30.687) -> (219.2863, -37.7893)
  line L152 (183.6, -59.4) -> (197.6, -59.4)
  line L153 (125.45, -74.65) -> (141.45, -74.65)
  circle A11 centre (76.6904, -49.9778) radius 2
  line L154 (99.2811, -148.0225) -> (98.1564, -148.3556)
  line L155 (218.4, -126.194) -> (179.1936, -126.194)
  line L156 (106.4, -61.05) -> (106.4, -77.05)
  line L157 (81.5052, -30.6903) -> (172.0779, -30.687)
  line L158 (178.55, -111.75) -> (178.55, -97.75)
  line L159 (75.7987, -35.5252) -> (76.1534, -34.3806)
  line L160 (93.1049, -146.6975) -> (92.4734, -145.8895)
  line L161 (224.2111, -122.2279) -> (223.6086, -123.3412)
  line L162 (135.898, -117.828) -> (135.898, -131.828)
  line L163 (159.5, -77.31) -> (145.5, -77.31)
  line L164 (130.85, -133.2) -> (130.85, -119.2)
  line L165 (116.85, -119.2) -> (116.85, -133.2)
  line L166 (224.1387, -42.1727) -> (224.705, -44.1568)
  line L167 (224.5766, -121.0472) -> (224.2111, -122.2279)
  line L168 (164.55, -54.6) -> (178.55, -54.6)
  line L169 (99.9784, -147.6695) -> (99.2811, -148.0225)
  line L170 (223.6086, -123.3412) -> (222.8109, -124.3089)
  line L171 (96.7866, -148.4476) -> (95.3567, -148.1592)
  line L172 (116.85, -133.2) -> (130.85, -133.2)
  line L173 (170.9399, -140.905) -> (111.6629, -140.905)
  line L174 (94.0822, -147.5328) -> (93.1049, -146.6975)
  line L175 (164.55, -97.75) -> (164.55, -111.75)
  line L176 (202.65, -85) -> (202.65, -99)
  line L177 (145.5, -77.31) -> (145.5, -91.31)
  line L178 (126.45, -73.65) -> (140.45, -73.65)
  line L179 (177.082, -135.7313) -> (176.7022, -136.9441)
  line L180 (107.4, -62.05) -> (107.4, -76.05)
  line L181 (77.4564, -32.4462) -> (78.3553, -31.7047)
  line L182 (130.85, -119.2) -> (116.85, -119.2)
  line L183 (107.4, -57) -> (121.4, -57)
  line L184 (76.7158, -33.3442) -> (77.4564, -32.4462)
  line L185 (223.044, -40.2889) -> (224.1387, -42.1727)
  line L186 (121.4, -43) -> (107.4, -43)
  line L187 (76.6839, -118.0469) -> (76.2792, -116.505)
  line L188 (75.7005, -36.4881) -> (75.7987, -35.5252)
  line L189 (121.4, -62.05) -> (107.4, -62.05)
  line L190 (171.9999, -140.8) -> (170.9399, -140.905)
  line L191 (121.4, -57) -> (121.4, -43)
  line L192 (75.9418, -114.8181) -> (75.7886, -113.0573)
  line L193 (98.23, -71.09) -> (98.23, -40.39)
  line L194 (75.7186, -112.1461) -> (75.6449, -110.7467)
  line L195 (175.3059, -139.0179) -> (174.3382, -139.8156)
  line L196 (216.65, -99) -> (216.65, -85)
  line L197 (107.4, -114.15) -> (121.4, -114.15)
  line L198 (176.7022, -136.9441) -> (176.1036, -138.0502)
  line L199 (145.5, -91.31) -> (159.5, -91.31)
  line L200 (98.1564, -148.3556) -> (96.7866, -148.4476)
  line L201 (219.4745, -126.0997) -> (218.4, -126.194)
  line L202 (178.55, -97.75) -> (164.55, -97.75)
  line L203 (107.4, -43) -> (107.4, -57)
  line L204 (76.1534, -34.3806) -> (76.7158, -33.3442)
  line L205 (177.193, -134.6953) -> (177.082, -135.7313)
  line L206 (85.03, -40.39) -> (85.03, -71.09)
  line L207 (164.55, -111.75) -> (178.55, -111.75)
  line L208 (95.3567, -148.1592) -> (94.0822, -147.5328)
  line L209 (178.55, -54.6) -> (178.55, -40.6)
  line L210 (222.8109, -124.3089) -> (221.8432, -125.1066)
  line L211 (126.45, -59.65) -> (126.45, -73.65)
  line L212 (164.55, -40.6) -> (164.55, -54.6)
  line L213 (216.65, -85) -> (202.65, -85)
  line L214 (178.55, -40.6) -> (164.55, -40.6)
  line L215 (77.5111, -119.9268) -> (76.6839, -118.0469)
  line L216 (140.45, -59.65) -> (126.45, -59.65)
  line L217 (202.65, -99) -> (216.65, -99)
  line L218 (98.23, -40.39) -> (85.03, -40.39)
  line L219 (221.8432, -125.1066) -> (220.7348, -125.7064)
  line L220 (107.4, -100.15) -> (107.4, -114.15)
  line L221 (159.5, -91.31) -> (159.5, -77.31)
  line L222 (121.4, -114.15) -> (121.4, -100.15)
  line L223 (121.4, -100.15) -> (107.4, -100.15)
  line L224 (135.898, -131.828) -> (149.898, -131.828)
  line L225 (220.7348, -125.7064) -> (219.4745, -126.0997)
  line L226 (85.03, -71.09) -> (98.23, -71.09)
  line L227 (149.898, -131.828) -> (149.898, -117.828)
  line L228 (140.45, -40.6) -> (126.45, -40.6)
  line L229 (126.45, -40.6) -> (126.45, -54.6)
  line L230 (140.45, -73.65) -> (140.45, -59.65)
  line L231 (75.7886, -113.0573) -> (75.7186, -112.1461)
  line L232 (149.898, -117.828) -> (135.898, -117.828)
  line L233 (140.45, -54.6) -> (140.45, -40.6)
  line L234 (216.65, -60.9) -> (216.65, -46.9)
  line L235 (140.45, -78.7) -> (126.45, -78.7)
  line L236 (126.45, -78.7) -> (126.45, -92.7)
  line L237 (126.45, -54.6) -> (140.45, -54.6)
  line L238 (126.45, -92.7) -> (140.45, -92.7)
  line L239 (159.5, -72.26) -> (159.5, -58.26)
  line L240 (159.5, -58.26) -> (145.5, -58.26)
  line L241 (145.5, -58.26) -> (145.5, -72.26)
  line L242 (145.5, -72.26) -> (159.5, -72.26)
  line L243 (178.55, -73.65) -> (178.55, -59.65)
  line L244 (178.55, -59.65) -> (164.55, -59.65)
  line L245 (164.55, -59.65) -> (164.55, -73.65)
  line L246 (183.6, -64.45) -> (183.6, -78.45)
  line L247 (216.65, -46.9) -> (202.65, -46.9)
  line L248 (202.65, -46.9) -> (202.65, -60.9)
  line L249 (202.65, -60.9) -> (216.65, -60.9)
  line L250 (140.45, -92.7) -> (140.45, -78.7)
  line L251 (164.55, -73.65) -> (178.55, -73.65)
  line L252 (197.6, -78.45) -> (197.6, -64.45)
  line L253 (183.6, -116.55) -> (197.6, -116.55)
  line L254 (183.6, -102.55) -> (183.6, -116.55)
  line L255 (97.4748, -105.2852) -> (97.4748, -91.2851)
  line L256 (197.6, -64.45) -> (183.6, -64.45)
  line L257 (197.6, -116.55) -> (197.6, -102.55)
  line L258 (83.4748, -105.2852) -> (97.4748, -105.2852)
  line L259 (97.4748, -91.2851) -> (83.4748, -91.2851)
  line L260 (219.259, -120.757) -> (219.037, -120.94)
  line L261 (219.037, -120.94) -> (218.782, -121.078)
  line L262 (81.7544, -35.6903) -> (171.704, -35.687)
  line L263 (81.9785, -117.665) -> (81.4197, -116.395)
  line L264 (80.772, -112.649) -> (80.7085, -111.823)
  line L265 (218.181, -121.194) -> (175.719, -121.194)
  line L266 (122.4, -99.15) -> (106.4, -99.15)
  line L267 (175.014, -121.265) -> (174.356, -121.468)
  line L268 (164.55, -78.7) -> (164.55, -92.7)
  line L269 (140.45, -97.75) -> (126.45, -97.75)
  line L270 (81.153, -115.379) -> (80.899, -114.109)
  line L271 (164.55, -92.7) -> (178.55, -92.7)
  line L272 (178.55, -92.7) -> (178.55, -78.7)
  line L273 (178.55, -78.7) -> (164.55, -78.7)
  line L274 (80.899, -114.109) -> (80.772, -112.649)
  line L275 (96.7353, -143.223) -> (96.6298, -143.088)
  line L276 (96.8523, -143.323) -> (96.7353, -143.223)
  line L277 (81.4197, -116.395) -> (81.153, -115.379)
  line L278 (80.645, -110.617) -> (80.7003, -36.7444)
  line L279 (80.7085, -111.823) -> (80.645, -110.617)
  line L280 (96.6298, -143.088) -> (81.9785, -117.665)
  line L281 (218.2905, -123.694) -> (177.6938, -123.694)
  arc A12 (177.6938, -123.694) -> (174.6938, -126.6937) centre (177.6938, -126.694) ccw
  line L282 (221.0885, -41.8996) -> (221.8203, -43.1589)
  line L283 (172.2545, -138.1006) -> (171.498, -138.3375)
  line L284 (80.8802, -36.1532) -> (81.0083, -35.9979)
  line L285 (218.782, -121.078) -> (218.5, -121.166)
  line L286 (172.193, -134.428) -> (172.163, -134.708)
  line L287 (217.796, -42.6214) -> (218.512, -42.9664)
  line L288 (97.2682, -143.404) -> (97.1193, -143.414)
  line L289 (172.817, -122.736) -> (172.494, -123.331)
  line L290 (218.512, -42.9664) -> (219.133, -43.5102)
  line L291 (97.1193, -143.414) -> (96.9805, -143.386)
  line L292 (96.9805, -143.386) -> (96.8523, -143.323)
  line L293 (110.32, -135.905) -> (97.5948, -143.272)
  line L294 (219.667, -119.999) -> (219.58, -120.28)
  line L295 (97.4269, -143.357) -> (97.2682, -143.404)
  line L296 (144.5, -95.36) -> (144.5, -111.36)
  line L297 (219.442, -120.535) -> (219.259, -120.757)
  line L298 (171.704, -35.687) -> (217.796, -42.6214)
  line L299 (144.5, -57.26) -> (144.5, -73.26)
  line L300 (80.7223, -36.5288) -> (80.7834, -36.3316)
  line L301 (219.502, -44.1452) -> (219.705, -44.8564)
  line L302 (125.45, -96.75) -> (125.45, -112.75)
  line L303 (219.58, -120.28) -> (219.442, -120.535)
  line L304 (81.1637, -35.8697) -> (81.3421, -35.773)
  line L305 (83.4748, -91.2851) -> (83.4748, -105.2852)
  arc A13 (80.8467, -125.7147) -> (89.7788, -141.2137) centre (86.1791, -132.9649) ccw
  line L306 (145.5, -96.36) -> (145.5, -110.36)
  arc A14 (75.6971, -41.0327) -> (75.6837, -58.9213) centre (76.6904, -49.9778) ccw
  arc A15 (224.704, -119.9944) -> (224.705, -102.1057) centre (223.705, -111.05) ccw
  line L307 (144.5, -76.31) -> (144.5, -92.31)
  line L308 (182.6, -98.5) -> (198.6, -98.5)
  line L309 (172.494, -123.331) -> (172.29, -123.988)
  line L310 (182.6, -82.5) -> (182.6, -98.5)
  line L311 (172.194, -124.696) -> (172.193, -134.428)
  line L312 (81.0083, -35.9979) -> (81.1637, -35.8697)
  line L313 (160.5, -76.31) -> (144.5, -76.31)
  line L314 (171.754, -135.466) -> (171.532, -135.649)
  line L315 (144.5, -73.26) -> (160.5, -73.26)
  line L316 (171.532, -135.649) -> (171.277, -135.787)
  line L317 (144.5, -111.36) -> (160.5, -111.36)
  line L318 (219.705, -119.685) -> (219.667, -119.999)
  line L319 (81.5392, -35.7118) -> (81.7544, -35.6903)
  line L320 (160.5, -111.36) -> (160.5, -95.36)
  line L321 (173.762, -121.791) -> (173.244, -122.218)
  line L322 (218.5, -121.166) -> (218.181, -121.194)
  line L323 (172.29, -123.988) -> (172.194, -124.696)
  line L324 (172.075, -134.989) -> (171.937, -135.244)
  line L325 (171.937, -135.244) -> (171.754, -135.466)
  line L326 (122.4, -115.15) -> (122.4, -99.15)
  line L327 (97.5948, -143.272) -> (97.4269, -143.357)
  line L328 (141.45, -96.75) -> (125.45, -96.75)
  line L329 (172.163, -134.708) -> (172.075, -134.989)
  line L330 (171.277, -135.787) -> (170.996, -135.875)
  line L331 (170.996, -135.875) -> (170.693, -135.905)
  line L332 (80.7834, -36.3316) -> (80.8802, -36.1532)
  line L333 (125.45, -112.75) -> (141.45, -112.75)
  line L334 (106.4, -99.15) -> (106.4, -115.15)
  line L335 (174.356, -121.468) -> (173.762, -121.791)
  line L336 (160.5, -57.26) -> (144.5, -57.26)
  line L337 (173.244, -122.218) -> (172.817, -122.736)
  line L338 (81.3421, -35.773) -> (81.5392, -35.7118)
  line L339 (80.7003, -36.7444) -> (80.7223, -36.5288)
  line L340 (160.5, -95.36) -> (144.5, -95.36)
  line L341 (160.5, -73.26) -> (160.5, -57.26)
  line L342 (219.133, -43.5102) -> (219.502, -44.1452)
  line L343 (175.719, -121.194) -> (175.014, -121.265)
  line L344 (141.45, -112.75) -> (141.45, -96.75)
  line L345 (170.693, -135.905) -> (110.32, -135.905)
  line L346 (106.4, -115.15) -> (122.4, -115.15)
  line L347 (219.705, -44.8564) -> (219.705, -119.685)
  line L348 (106.4, -96.1) -> (122.4, -96.1)
  line L349 (179.55, -112.75) -> (179.55, -96.75)
  line L350 (201.65, -80.95) -> (217.65, -80.95)
  line L351 (106.4, -80.1) -> (106.4, -96.1)
  line L352 (163.55, -112.75) -> (179.55, -112.75)
  line L353 (182.6, -79.45) -> (198.6, -79.45)
  line L354 (179.55, -96.75) -> (163.55, -96.75)
  line L355 (197.6, -97.5) -> (197.6, -83.5)
  line L356 (160.5, -92.31) -> (160.5, -76.31)
  line L357 (198.6, -117.55) -> (198.6, -101.55)
  line L358 (182.6, -117.55) -> (198.6, -117.55)
  line L359 (122.4, -80.1) -> (106.4, -80.1)
  line L360 (163.55, -96.75) -> (163.55, -112.75)
  line L361 (122.4, -96.1) -> (122.4, -80.1)
  line L362 (144.5, -92.31) -> (160.5, -92.31)
  line L363 (163.55, -93.7) -> (179.55, -93.7)
  line L364 (183.6, -83.5) -> (183.6, -97.5)
  line L365 (163.55, -58.65) -> (163.55, -74.65)
  line L366 (141.45, -93.7) -> (141.45, -77.7)
  line L367 (94.9201, -144.9603) -> (94.5516, -144.4887)
  line L368 (79.7448, -118.7959) -> (79.0518, -117.2209)
  line L369 (218.5412, -40.2054) -> (219.9033, -40.8617)
  line L370 (96.1686, -145.7726) -> (95.4672, -145.4279)
  arc A16 (90.6367, -137.6956) -> (84.3208, -126.7362) centre (86.1791, -132.9649) cw
  line L371 (84.3208, -126.7362) -> (79.7448, -118.7959)
  line L372 (150.898, -116.828) -> (134.898, -116.828)
  line L373 (95.4672, -145.4279) -> (94.9201, -144.9603)
  line L374 (98.7866, -145.4708) -> (98.354, -145.6898)
  line L375 (173.5299, -137.2419) -> (172.9351, -137.7323)
  line L376 (101.0994, -115.1193) -> (87.243, -123.1193)
  line L377 (78.7161, -115.942) -> (78.4204, -114.4636)
  line L378 (78.4204, -114.4636) -> (78.2803, -112.8531)
  line L379 (79.0518, -117.2209) -> (78.7161, -115.942)
  line L380 (174.3886, -135.9665) -> (174.0203, -136.6471)
  line L381 (222.205, -44.5066) -> (222.205, -47.5754)
  line L382 (78.2803, -112.8531) -> (78.2135, -111.9846)
  line L383 (94.5516, -144.4887) -> (90.6367, -137.6956)
  line L384 (78.2135, -111.9846) -> (78.145, -110.6818)
  line L385 (88.03, -43.39) -> (88.03, -68.09)
  line L386 (97.7123, -145.8798) -> (96.953, -145.9308)
  line L387 (222.1218, -120.5231) -> (221.8955, -121.2539)
  line L388 (153.95, -115.8) -> (153.95, -131.8)
  line L389 (134.898, -132.828) -> (150.898, -132.828)
  line L390 (219.9033, -40.8617) -> (221.0885, -41.8996)
  line L391 (221.8955, -121.2539) -> (221.5253, -121.9381)
  line L392 (218.9873, -123.6328) -> (218.2905, -123.694)
  line L393 (174.6938, -126.6937) -> (174.693, -134.5617)
  line L394 (131.85, -134.2) -> (131.85, -118.2)
  line L395 (110.9915, -138.405) -> (98.7866, -145.4708)
  line L396 (221.0349, -122.5329) -> (220.4401, -123.0233)
  line L397 (88.03, -68.09) -> (95.23, -68.09)
  arc A17 (222.205, -47.5754) -> (222.205, -60.2246) centre (223.705, -53.9) cw
  line L398 (174.693, -134.5617) -> (174.6225, -135.2197)
  line L399 (172.9351, -137.7323) -> (172.2545, -138.1006)
  line L400 (96.953, -145.9308) -> (96.1686, -145.7726)
  line L401 (109.0994, -128.9757) -> (101.0994, -115.1193)
  line L402 (95.243, -136.9757) -> (109.0994, -128.9757)
  line L403 (221.5253, -121.9381) -> (221.0349, -122.5329)
  line L404 (98.354, -145.6898) -> (97.7123, -145.8798)